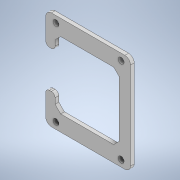
# Autodesk Inventor part: wood_supp
Saved by Autodesk Inventor 2021 (Build 250183000, 183)
## iProperties
Created: 2023-10-27
Part Number: wood_supp
Material: Generic
Document SubType Name: Modeling
Designer: Toby
Density: 1 g/cm^3
Appearance: Default
Author: Toby
Autodesk Inventor part; units mm, degrees
ref_plane "YZ Plane" through (0, 0, 0) normal (1, 0, 0) x (0, 1, 0)
ref_plane "XZ Plane" through (0, 0, 0) normal (0, 1, 0) x (-1, 0, 0)
ref_plane "XY Plane" through (0, 0, 0) normal (0, 0, 1) x (1, 0, 0)
sketch "Sketch1" plane through (0, 0, 0) normal (0, 0, 1) x (1, 0, 0)
  line L0 (-18.671, 23.6638) -> (26.829, 23.6638)
  line L1 (26.829, 23.6638) -> (26.829, -28.3362)
  line L2 (26.829, -28.3362) -> (-18.671, -28.3362)
  line L3 (-18.671, -28.3362) -> (-18.671, 23.6638)
  point P0 (0, 0)
  dimension "d0" = 52
  dimension "d1" = 45.5
  constraints: 8 end point, 2 parallel, 1 horizontal, 1 perpendicular
  measures "d0" distance of L0.end L1.end
  measures "d1" distance of L0.start L0.end
extrude "Extrusion1" add sketch "Sketch1" along normal blind 2
sketch "Sketch2" plane through (0, 0, 2) normal (0, 0, 1) x (1, 0, 0)
  line L0 (-18.671, -28.3362) -> (26.829, -28.3362) projected
  line L1 (26.829, -28.3362) -> (26.829, 23.6638) projected
  line L2 (26.829, 23.6638) -> (-18.671, 23.6638) projected
  point P0 (0, 0)
  point P1 (-13.171, 20.6638)
  point P2 (21.829, 20.6638)
  point P3 (21.829, -25.3362)
  point P4 (-13.171, -25.3362)
  point P5 (23.829, -28.3362)
  point P6 (26.829, -25.3362)
  point P7 (26.829, 20.6638)
  point P8 (23.829, 23.6638)
  dimension "d5" = 35
  dimension "d6" = 35
  dimension "d7" = 46
  dimension "d8" = 3
  dimension "d9" = 3
  dimension "d10" = 5
  dimension "d11" = 5
  dimension "d12" = 3
  measures "d5" distance of point (21.829, 20.664) point (-13.171, 20.664)
  measures "d6" distance of point (21.829, -25.336) point (-13.171, -25.336)
  measures "d7" distance of point (21.829, 20.664) point (21.829, -25.336)
  measures "d8" distance from line of L0 point (-13.171, -25.336)
  measures "d9" distance from line of L0 point (21.829, -25.336)
  measures "d10" distance from line of L1 point (21.829, 20.664)
  measures "d11" distance from line of L1 point (21.829, -25.336)
  measures "d12" distance from line of L2 point (-13.171, 20.664)
hole "Hole1" at (-13.171, 20.6638, 2) at (21.829, 20.6638, 2) at (21.829, -25.3362, 2) at (-13.171, -25.3362, 2) direction (0, 0, -1) diameter 3.2 depth 10 tip angle 118
sketch "Sketch3" plane through (0, 0, 2) normal (0, 0, 1) x (1, 0, 0)
  line L0 (-18.671, 23.6638) -> (-18.671, -28.3362) projected
  line L1 (-18.671, 15.6638) -> (20.829, 15.6638)
  line L2 (20.829, 15.6638) -> (20.829, -20.3362)
  line L3 (20.829, -20.3362) -> (-18.671, -20.3362)
  line L4 (-18.671, -20.3362) -> (-18.671, 15.6638)
  circle A0 centre (-13.171, 20.6638) radius 1.6 projected
  line L5 (26.829, -28.3362) -> (26.829, 23.6638) projected
  circle A1 centre (-13.171, -25.3362) radius 1.6 projected
  point P0 (0, 0)
  point P1 (26.829, -25.3362)
  point P2 (26.829, 20.6638)
  dimension "d20" = 5
  dimension "d21" = 6
  dimension "d22" = 5
  constraints: 8 end point, 2 parallel, 1 horizontal, 1 perpendicular, 1 point on line
  measures "d20" distance from line of L1 A0.centre
  measures "d21" distance between parallel lines of L5 L2
  measures "d22" distance from line of A1.centre L3
extrude "Extrusion2" cut sketch "Sketch3" against normal blind 2 contours L1 L2 L3 L0
sketch "Sketch4" plane through (0, 0, 2) normal (0, 0, 1) x (1, 0, 0)
  line L0 (-18.671, 15.6638) -> (20.829, 15.6638) projected
  line L1 (-18.671, 15.6638) -> (-13.671, 15.6638)
  line L2 (-13.671, 15.6638) -> (-13.671, 7.6638)
  line L3 (-13.671, 7.6638) -> (-18.671, 7.6638)
  line L4 (-18.671, 7.6638) -> (-18.671, 15.6638)
  line L5 (-18.671, -20.3362) -> (-18.671, -28.3362) projected
  line L6 (-18.671, -20.3362) -> (-13.671, -20.3362)
  line L7 (-13.671, -20.3362) -> (-13.671, -12.3362)
  line L8 (-13.671, -12.3362) -> (-18.671, -12.3362)
  line L9 (-18.671, -12.3362) -> (-18.671, -20.3362)
  point P0 (0, 0)
  point P1 (17.829, 15.6638)
  point P2 (-18.671, -25.3362)
  dimension "d27" = 8
  dimension "d28" = 8
  dimension "d29" = 5
  constraints: 16 end point, 4 parallel, 2 horizontal, 2 perpendicular, 1 point on line
  measures "d27" distance between parallel lines of L0 L3
  measures "d28" distance between parallel lines of L6 L8
  measures "d29" distance between parallel lines of L4 L2
extrude "Extrusion3" add sketch "Sketch4" against normal blind 2
fillet "Fillet5" radius 2 4 edges at (-13.671, 7.6638, 1) (-18.671, 7.6638, 1) (-18.671, -12.3362, 1) (-13.671, -12.3362, 1)
sketch "Sketch5" plane through (0, 0, 2) normal (0, 0, 1) x (1, 0, 0)
  line L0 (26.829, 23.6638) -> (-18.671, 23.6638) projected
  line L1 (-18.671, 23.6638) -> (26.829, 23.6638)
  line L2 (26.829, 23.6638) -> (26.829, 24.1638)
  line L3 (26.829, 24.1638) -> (-18.671, 24.1638)
  line L4 (-18.671, 24.1638) -> (-18.671, 23.6638)
  line L5 (-18.671, -28.3362) -> (26.829, -28.3362) projected
  line L6 (-18.671, -28.3362) -> (26.829, -28.3362)
  line L7 (26.829, -28.3362) -> (26.829, -28.8362)
  line L8 (26.829, -28.8362) -> (-18.671, -28.8362)
  line L9 (-18.671, -28.8362) -> (-18.671, -28.3362)
  line L10 (26.829, -28.3362) -> (26.829, 23.6638) projected
  point P0 (0, 0)
  dimension "d37" = 0.5
  dimension "d38" = 0.5
  constraints: 16 end point, 4 parallel, 2 horizontal, 2 perpendicular, 1 collinear, 1 point on line
  measures "d37" distance between parallel lines of L0 L3
  measures "d38" distance between parallel lines of L5 L8
extrude "Extrusion4" add sketch "Sketch5" against normal blind 2
fillet "Fillet6" radius 3 4 edges at (-18.671, 24.1638, 1) (26.829, 24.1638, 1) (26.829, -28.8362, 1) (-18.671, -28.8362, 1)
chamfer "Chamfer2" distance 3 angle 45 4 edges at (-13.671, 15.6638, 1) (20.829, 15.6638, 1) (-13.671, -20.3362, 1) (20.829, -20.3362, 1)
body "Solid1"
